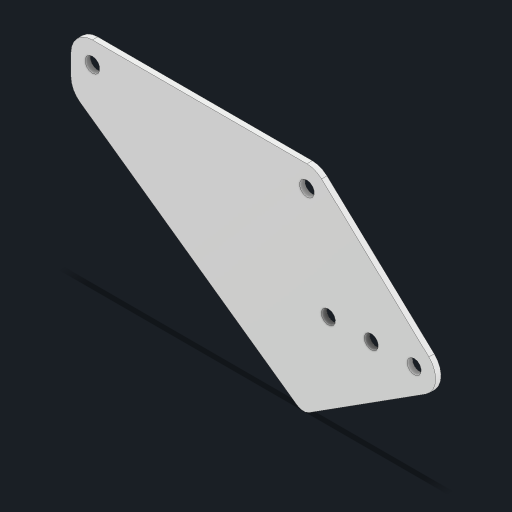
# Autodesk Inventor part: sled
Saved by Autodesk Inventor 2024 (Build 280153000, 153)
## iProperties
Created: 2024-03-05
Part Number: sled
Material: Acetal Resin, White
Document SubType Name: Modeling
Designer: Averey Ku
Density: 1.425 g/cm^3
Appearance: Smooth - White
Author: Averey Ku
Autodesk Inventor part; units mm, degrees
ref_plane "YZ Plane" through (0, 0, 0) normal (1, 0, 0) x (0, 1, 0)
ref_plane "XZ Plane" through (0, 0, 0) normal (0, 1, 0) x (-1, 0, 0)
ref_plane "XY Plane" through (0, 0, 0) normal (0, 0, 1) x (1, 0, 0)
sketch "main" plane through (0, 0, 0) normal (0, 0, 1) x (1, 0, 0)
  line L0 (10.9249, 53.4086) -> (-34.6395, -10.8755)
  line L1 (28.7127, 49.7366) -> (28.7127, -13.7634)
  arc A0 (16.1055, 56.0866) -> (10.9249, 53.4086) centre (16.1055, 49.7366) ccw
  line L2 (22.3627, 56.0866) -> (16.1055, 56.0866)
  arc A1 (28.7127, 49.7366) -> (22.3627, 56.0866) centre (22.3627, 49.7366) ccw
  arc A2 (26.9969, -18.1047) -> (28.7127, -13.7634) centre (22.3627, -13.7634) ccw
  arc A3 (-34.6395, -10.8755) -> (-34.7267, -14.4179) centre (-32.0492, -12.7116) ccw
  line L3 (-2.7465, -49.8547) -> (26.9969, -18.1047)
  circle A4 centre (-7.3807, -45.5134) radius 2.0955
  arc A5 (-12.7358, -48.926) -> (-2.7465, -49.8547) centre (-7.3807, -45.5134) ccw
  line L4 (-34.7267, -14.4179) -> (-12.7358, -48.926)
  circle A6 centre (-7.3807, -20.1134) radius 2.0955
  circle A7 centre (22.3627, 49.7366) radius 2.1844
  circle A8 centre (22.3627, -13.7634) radius 2.1844
  circle A9 centre (-7.3807, -32.8134) radius 2.0955
  point P0 (3.7494, 2.3687)
  point P1 (14.8443, 56.0866)
  dimension "d0" = 6.35
  dimension "d1" = 4.191
  dimension "d2" = 12.7
  dimension "d3" = 3.175
  dimension "d4" = 4.3688
  dimension "d5" = 4.3688
  dimension "d6" = 4.191
  dimension "d7" = 4.191
  measures "d0" radius of A0
  measures "d1" diameter of A4
  measures "d2" diameter of A5
  measures "d3" radius of A3
  measures "d4" diameter of A7
  measures "d5" diameter of A8
  measures "d6" diameter of A9
  measures "d7" diameter of A6
sketch "Sketch1" plane through (0, 0, 0) normal (0, 0, 1) x (1, 0, 0)
  line L0 (-73.522, 18.3056) -> (-9.2379, -27.2588)
  line L1 (-69.85, 36.0934) -> (-6.35, 36.0934)
  arc A0 (-76.2, 23.4862) -> (-73.522, 18.3056) centre (-69.85, 23.4862) ccw
  line L2 (-76.2, 29.7434) -> (-76.2, 23.4862)
  arc A1 (-69.85, 36.0934) -> (-76.2, 29.7434) centre (-69.85, 29.7434) ccw
  arc A2 (-2.0087, 34.3776) -> (-6.35, 36.0934) centre (-6.35, 29.7434) ccw
  arc A3 (-9.2379, -27.2588) -> (-5.6956, -27.346) centre (-7.4019, -24.6685) ccw
  line L3 (29.7413, 4.6342) -> (-2.0087, 34.3776)
  circle A4 centre (25.4, 0) radius 2.0955
  arc A5 (28.8126, -5.3551) -> (29.7413, 4.6342) centre (25.4, 0) ccw
  line L4 (-5.6956, -27.346) -> (28.8126, -5.3551)
  circle A6 centre (0, 0) radius 2.0955
  circle A7 centre (-69.85, 29.7434) radius 2.1844
  circle A8 centre (-6.35, 29.7434) radius 2.1844
  circle A9 centre (12.7, 0) radius 2.0955
  constraints: 1 other
extrude "Extrusion1" add sketch "Sketch1" along normal blind 1.5875
body "Solid1"
